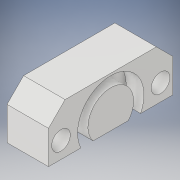
# Autodesk Inventor part: Spreader Holder
Saved by Autodesk Inventor 2018 (Build 220112000, 112)
## iProperties
Created: 2014-02-15
Part Number: Spreader Holder
Material: ASA Plastic
Document SubType Name: Modeling
Designer: Gabriel Smolnycki
Mass: 3.01167 g
Surface Area: 19.2103 cm^2
Volume: 2.81465 cm^3
Density: 1.07 g/cm^3
Appearance: Smooth - White ASA
Sending System: SolidWorks 2017
Last Author: Gabriel Smolnycki
Last Saved: 2017-09-14
Author: Gabriel Smolnycki
Autodesk Inventor part; units mm, degrees
ref_plane "YZ Plane" through (0, 0, 0) normal (1, 0, 0) x (0, 1, 0)
ref_plane "XZ Plane" through (0, 0, 0) normal (0, 1, 0) x (-1, 0, 0)
ref_plane "XY Plane" through (0, 0, 0) normal (0, 0, 1) x (1, 0, 0)
sketch "Sketch1" plane through (0, 0, 0) normal (1, 0, 0) x (0, 1, 0)
  line L0 (12, 11) -> (8, 15)
  line L1 (8, 15) -> (0, 15)
  line L2 (0, 15) -> (0, -15)
  line L3 (8, -15) -> (12, -11)
  line L4 (12, -11) -> (12, 11)
  line L5 (0, -15) -> (8, -15)
  constraints: 12 end point, 2 equal length, 2 horizontal, 2 vertical, 1 perpendicular
extrude "Extrusion2" add sketch "Sketch1" along normal blind 10
sketch "Sketch2" plane through (10, 0, 0) normal (1, 0, 0) x (0, 0, -1)
  line L0 (4.2426, 0) -> (7.1937, 0)
  arc A0 (4.2426, 0) -> (-4.2426, 0) centre (0, 3.5) ccw
  arc A1 (7.1937, 0) -> (-7.1937, 0) centre (0, 3.5) ccw
  line L1 (-7.1937, 0) -> (-4.2426, 0)
  constraints: 4 end point, 4 point on circle, 2 centre point, 2 collinear, 2 horizontal
extrude "Extrusion1" cut sketch "Sketch2" against normal blind 4.3
hole "Hole2" at (0, 4, -12) direction (1, 0, 0) diameter 4.5 depth 10 tip angle 118
sketch "Sketch3" plane through (0, 0, 0) normal (1, 0, 0) x (0, 1, 0)
  point P0 (4, -12)
hole "Hole1" at (0, 4, 12) direction (1, 0, 0) diameter 4.5 depth 10 tip angle 118
sketch "Sketch4" plane through (0, 0, 0) normal (1, 0, 0) x (0, 1, 0)
  point P0 (4, 12)
body "Solid3"
